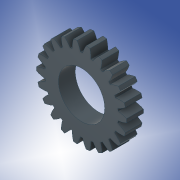
# Autodesk Inventor part: Motor Coupler
Saved by Autodesk Inventor 2017 SP1 (Build 210196100, 196)
## iProperties
Created: 2017-07-05
Part Number: Motor Coupler
Material: ABS Plastic
Document SubType Name: Modeling
Designer: zallen
Density: 1.06 g/cm^3
Appearance: CR Dark Blue
Author: zallen
Autodesk Inventor part; units mm, degrees
ref_plane "YZ Plane" through (0, 0, 0) normal (1, 0, 0) x (0, 1, 0)
ref_plane "XZ Plane" through (0, 0, 0) normal (0, 1, 0) x (-1, 0, 0)
ref_plane "XY Plane" through (0, 0, 0) normal (0, 0, 1) x (1, 0, 0)
sketch "Sketch1" plane through (0, 0, 0) normal (0, 0, 1) x (1, 0, 0)
  circle A0 centre (0, 0) radius 17.5
  dimension "d0" = 35
  constraints: 1 centre point, 1 coincident
  measures "d0" diameter of A0
extrude "Extrusion1" add sketch "Sketch1" along normal blind 8
sketch "Sketch7" plane through (0, 0, 8) normal (0, 0, 1) x (1, 0, 0)
  circle A0 centre (0, 0) radius 17.5 construction
  line L0 (0, 0) -> (15, 0) construction
  circle A1 centre (0, 0) radius 17.5 projected
  arc A2 (21.3853, 0.9) -> (17.3853, 2) centre (15.4462, -12.8741) ccw
  arc A3 (21.3853, -0.9) -> (21.3853, 0.9) centre (1.4056, 0) ccw
  arc A4 (17.3853, -2) -> (21.3853, -0.9) centre (15.4462, 12.8741) ccw
  arc A5 (17.3853, -2) -> (17.3853, 2) centre (0, 0) ccw
  arc A6 (20.2655, 6.8885) -> (16.1176, 6.817) centre (18.4476, -8.0009) ccw
  arc A7 (17.2446, 2.979) -> (16.1176, 6.817) centre (0, 0) ccw
  arc A8 (17.2446, 2.979) -> (20.7726, 5.1614) centre (11.1935, 16.7043) ccw
  arc A9 (20.7726, 5.1614) -> (20.2655, 6.8885) centre (1.3487, 0.396) ccw
  arc A10 (17.5039, 12.3189) -> (13.5442, 11.0817) centre (19.9545, -2.4796) ccw
  arc A11 (15.7068, 7.7167) -> (13.5442, 11.0817) centre (0, 0) ccw
  arc A12 (15.7068, 7.7167) -> (18.4771, 10.8047) centre (6.0339, 19.1813) ccw
  arc A13 (18.4771, 10.8047) -> (17.5039, 12.3189) centre (1.1825, 0.7599) ccw
  arc A14 (13.3242, 16.7513) -> (9.8735, 14.4487) centre (19.8447, 3.2427) ccw
  arc A15 (12.8965, 11.8292) -> (9.8735, 14.4487) centre (0, 0) ccw
  arc A16 (12.8965, 11.8292) -> (14.6846, 15.5726) centre (0.3855, 20.1042) ccw
  arc A17 (14.6846, 15.5726) -> (13.3242, 16.7513) centre (0.9205, 1.0623) ccw
  arc A18 (8.0651, 19.8267) -> (5.4029, 16.6451) centre (18.1273, 8.7023) ccw
  arc A19 (9.0414, 14.9834) -> (5.4029, 16.6451) centre (0, 0) ccw
  arc A20 (9.0414, 14.9834) -> (9.7025, 19.0789) centre (-5.2941, 19.3985) ccw
  arc A21 (9.7025, 19.0789) -> (8.0651, 19.8267) centre (0.5839, 1.2786) ccw
  arc A22 (2.1526, 21.2958) -> (0.4945, 17.493) centre (14.9413, 13.4568) ccw
  arc A23 (4.4538, 16.9238) -> (0.4945, 17.493) centre (0, 0) ccw
  arc A24 (4.4538, 16.9238) -> (3.9343, 21.0396) centre (-10.5449, 17.1212) ccw
  arc A25 (3.9343, 21.0396) -> (2.1526, 21.2958) centre (0.2, 1.3913) ccw
  arc A26 (-3.9343, 21.0396) -> (-4.4538, 16.9238) centre (10.5449, 17.1212) ccw
  arc A27 (-0.4945, 17.493) -> (-4.4538, 16.9238) centre (0, 0) ccw
  arc A28 (-0.4945, 17.493) -> (-2.1526, 21.2958) centre (-14.9413, 13.4568) ccw
  arc A29 (-2.1526, 21.2958) -> (-3.9343, 21.0396) centre (-0.2, 1.3913) ccw
  arc A30 (-9.7025, 19.0789) -> (-9.0414, 14.9834) centre (5.2941, 19.3985) ccw
  arc A31 (-5.4029, 16.6451) -> (-9.0414, 14.9834) centre (0, 0) ccw
  arc A32 (-5.4029, 16.6451) -> (-8.0651, 19.8267) centre (-18.1273, 8.7023) ccw
  arc A33 (-8.0651, 19.8267) -> (-9.7025, 19.0789) centre (-0.5839, 1.2786) ccw
  arc A34 (-14.6846, 15.5726) -> (-12.8965, 11.8292) centre (-0.3855, 20.1042) ccw
  arc A35 (-9.8735, 14.4487) -> (-12.8965, 11.8292) centre (0, 0) ccw
  arc A36 (-9.8735, 14.4487) -> (-13.3242, 16.7513) centre (-19.8447, 3.2427) ccw
  arc A37 (-13.3242, 16.7513) -> (-14.6846, 15.5726) centre (-0.9205, 1.0623) ccw
  arc A38 (-18.4771, 10.8047) -> (-15.7068, 7.7167) centre (-6.0339, 19.1813) ccw
  arc A39 (-13.5442, 11.0817) -> (-15.7068, 7.7167) centre (0, 0) ccw
  arc A40 (-13.5442, 11.0817) -> (-17.5039, 12.3189) centre (-19.9545, -2.4796) ccw
  arc A41 (-17.5039, 12.3189) -> (-18.4771, 10.8047) centre (-1.1825, 0.7599) ccw
  arc A42 (-20.7726, 5.1614) -> (-17.2446, 2.979) centre (-11.1935, 16.7043) ccw
  arc A43 (-16.1176, 6.817) -> (-17.2446, 2.979) centre (0, 0) ccw
  arc A44 (-16.1176, 6.817) -> (-20.2655, 6.8885) centre (-18.4476, -8.0009) ccw
  arc A45 (-20.2655, 6.8885) -> (-20.7726, 5.1614) centre (-1.3487, 0.396) ccw
  arc A46 (-21.3853, -0.9) -> (-17.3853, -2) centre (-15.4462, 12.8741) ccw
  arc A47 (-17.3853, 2) -> (-17.3853, -2) centre (0, 0) ccw
  arc A48 (-17.3853, 2) -> (-21.3853, 0.9) centre (-15.4462, -12.8741) ccw
  arc A49 (-21.3853, 0.9) -> (-21.3853, -0.9) centre (-1.4056, 0) ccw
  arc A50 (-20.2655, -6.8885) -> (-16.1176, -6.817) centre (-18.4476, 8.0009) ccw
  arc A51 (-17.2446, -2.979) -> (-16.1176, -6.817) centre (0, 0) ccw
  arc A52 (-17.2446, -2.979) -> (-20.7726, -5.1614) centre (-11.1935, -16.7043) ccw
  arc A53 (-20.7726, -5.1614) -> (-20.2655, -6.8885) centre (-1.3487, -0.396) ccw
  arc A54 (-17.5039, -12.3189) -> (-13.5442, -11.0817) centre (-19.9545, 2.4796) ccw
  arc A55 (-15.7068, -7.7167) -> (-13.5442, -11.0817) centre (0, 0) ccw
  arc A56 (-15.7068, -7.7167) -> (-18.4771, -10.8047) centre (-6.0339, -19.1813) ccw
  arc A57 (-18.4771, -10.8047) -> (-17.5039, -12.3189) centre (-1.1825, -0.7599) ccw
  arc A58 (-13.3242, -16.7513) -> (-9.8735, -14.4487) centre (-19.8447, -3.2427) ccw
  arc A59 (-12.8965, -11.8292) -> (-9.8735, -14.4487) centre (0, 0) ccw
  arc A60 (-12.8965, -11.8292) -> (-14.6846, -15.5726) centre (-0.3855, -20.1042) ccw
  arc A61 (-14.6846, -15.5726) -> (-13.3242, -16.7513) centre (-0.9205, -1.0623) ccw
  arc A62 (-8.0651, -19.8267) -> (-5.4029, -16.6451) centre (-18.1273, -8.7023) ccw
  arc A63 (-9.0414, -14.9834) -> (-5.4029, -16.6451) centre (0, 0) ccw
  arc A64 (-9.0414, -14.9834) -> (-9.7025, -19.0789) centre (5.2941, -19.3985) ccw
  arc A65 (-9.7025, -19.0789) -> (-8.0651, -19.8267) centre (-0.5839, -1.2786) ccw
  arc A66 (-2.1526, -21.2958) -> (-0.4945, -17.493) centre (-14.9413, -13.4568) ccw
  arc A67 (-4.4538, -16.9238) -> (-0.4945, -17.493) centre (0, 0) ccw
  arc A68 (-4.4538, -16.9238) -> (-3.9343, -21.0396) centre (10.5449, -17.1212) ccw
  arc A69 (-3.9343, -21.0396) -> (-2.1526, -21.2958) centre (-0.2, -1.3913) ccw
  arc A70 (3.9343, -21.0396) -> (4.4538, -16.9238) centre (-10.5449, -17.1212) ccw
  arc A71 (0.4945, -17.493) -> (4.4538, -16.9238) centre (0, 0) ccw
  arc A72 (0.4945, -17.493) -> (2.1526, -21.2958) centre (14.9413, -13.4568) ccw
  arc A73 (2.1526, -21.2958) -> (3.9343, -21.0396) centre (0.2, -1.3913) ccw
  arc A74 (9.7025, -19.0789) -> (9.0414, -14.9834) centre (-5.2941, -19.3985) ccw
  arc A75 (5.4029, -16.6451) -> (9.0414, -14.9834) centre (0, 0) ccw
  arc A76 (5.4029, -16.6451) -> (8.0651, -19.8267) centre (18.1273, -8.7023) ccw
  arc A77 (8.0651, -19.8267) -> (9.7025, -19.0789) centre (0.5839, -1.2786) ccw
  arc A78 (14.6846, -15.5726) -> (12.8965, -11.8292) centre (0.3855, -20.1042) ccw
  arc A79 (9.8735, -14.4487) -> (12.8965, -11.8292) centre (0, 0) ccw
  arc A80 (9.8735, -14.4487) -> (13.3242, -16.7513) centre (19.8447, -3.2427) ccw
  arc A81 (13.3242, -16.7513) -> (14.6846, -15.5726) centre (0.9205, -1.0623) ccw
  arc A82 (18.4771, -10.8047) -> (15.7068, -7.7167) centre (6.0339, -19.1813) ccw
  arc A83 (13.5442, -11.0817) -> (15.7068, -7.7167) centre (0, 0) ccw
  arc A84 (13.5442, -11.0817) -> (17.5039, -12.3189) centre (19.9545, 2.4796) ccw
  arc A85 (17.5039, -12.3189) -> (18.4771, -10.8047) centre (1.1825, -0.7599) ccw
  arc A86 (20.7726, -5.1614) -> (17.2446, -2.979) centre (11.1935, -16.7043) ccw
  arc A87 (16.1176, -6.817) -> (17.2446, -2.979) centre (0, 0) ccw
  arc A88 (16.1176, -6.817) -> (20.2655, -6.8885) centre (18.4476, 8.0009) ccw
  arc A89 (20.2655, -6.8885) -> (20.7726, -5.1614) centre (1.3487, -0.396) ccw
  point P0 (21.4056, 0)
  point P1 (20.5385, 6.0307)
  point P2 (18.0075, 11.5727)
  point P3 (14.0177, 16.1773)
  point P4 (8.8922, 19.4712)
  point P5 (3.0463, 21.1877)
  point P6 (-3.0463, 21.1877)
  point P7 (-8.8922, 19.4712)
  point P8 (-14.0177, 16.1773)
  point P9 (-18.0075, 11.5727)
  point P10 (-20.5385, 6.0307)
  point P11 (-21.4056, 0)
  point P12 (-20.5385, -6.0307)
  point P13 (-18.0075, -11.5727)
  point P14 (-14.0177, -16.1773)
  point P15 (-8.8922, -19.4712)
  point P16 (-3.0463, -21.1877)
  point P17 (3.0463, -21.1877)
  point P18 (8.8922, -19.4712)
  point P19 (14.0177, -16.1773)
  point P20 (18.0075, -11.5727)
  point P21 (20.5385, -6.0307)
  dimension "d19" = 15
  dimension "d20" = 15
  dimension "d21" = 20
  dimension "d22" = 1.8
  dimension "d23" = 2
  dimension "d24" = 4
  dimension "d27" = 360
  constraints: 177 point on circle, 88 centre point, 2 end point, 2 symmetric about line, 1 horizontal, 1 point on line, 293 other
  measures "d19" distance of L0.start L0.end
  measures "d20" radius of A2
  measures "d21" radius of A3
  measures "d22" distance of A3.start A2.start
  measures "d23" distance from line of L0 A2.end
  measures "d24" horizontal distance of A2.end A2.start
extrude "Extrusion7" add sketch "Sketch7" against normal blind 8 contours A1 A2 A3 A4 | A1 A6 A9 A8 | A86 A89 A88 A1 | A1 A10 A13 A12 | A82 A85 A84 A1 | A1 A14 A17 A16 | A78 A81 A80 A1 | A1 A18 A21 A20 | A74 A77 A76 A1 | A1 A22 A25 A24 | A70 A73 A72 A1 | A1 A26 A29 A28 | A66 A69 A68 A1 | A1 A30 A33 A32 | A62 A65 A64 A1 | A1 A34 A37 A36 | A58 A61 A60 A1 | A1 A38 A41 A40 | A54 A57 A56 A1 | A1 A42 A45 A44 | A50 A53 A52 A1 | A1 A46 A49 A48
sketch "Sketch9" plane through (0, 0, 8) normal (0, 0, 1) x (1, 0, 0)
  circle A0 centre (0, 0) radius 11
  dimension "d33" = 22
  constraints: 1 centre point, 1 coincident
  measures "d33" diameter of A0
extrude "Extrusion9" cut sketch "Sketch9" against normal through all
body "Solid1"
